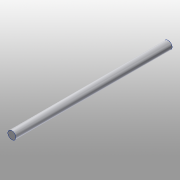
# Autodesk Inventor part: 500-169
Saved by Autodesk Inventor 2016 (Build 200138000, 138)
## iProperties
Created: 2015-04-18
Part Number: 500-169
Material: Aluminum 6061
Document SubType Name: Modeling
Designer: Station9
Density: 2.7 g/cm^3
Appearance: Aluminum - Flat
Mass: 1.12603 g
Surface Area: 5.70199 cm^2
Volume: 0.417046 cm^3
Author: Station9
Autodesk Inventor part; units mm, degrees
ref_plane "YZ Plane" through (0, 0, 0) normal (1, 0, 0) x (0, 1, 0)
ref_plane "XZ Plane" through (0, 0, 0) normal (0, 1, 0) x (-1, 0, 0)
ref_plane "XY Plane" through (0, 0, 0) normal (0, 0, 1) x (1, 0, 0)
sketch "Sketch1" plane through (0, 0, 0) normal (0, 1, 0) x (-1, 0, 0)
  circle A0 centre (0, 0) radius 1.5
  dimension "d0" = 3
  constraints: 1 centre point, 1 coincident
  measures "d0" diameter of A0
extrude "Extrusion1" add sketch "Sketch1" along normal blind 59
body "Solid1"
